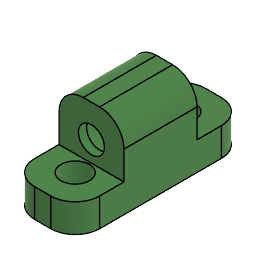
ServoTensioner_v2 (Autodesk Fusion 360 design; units mm, degrees)
Autodesk Fusion 360 part; units mm, degrees
sketch "Sketch1" plane through (0, 0, 0) normal (0, 0, 1) x (1, 0, 0)
  line L0 (0, 6.5) -> (0, -6.5) construction
  circle A0 centre (0, 6.5) radius 1.75
  circle A1 centre (0, -6.5) radius 1.75
  line L1 (4, -4.5) -> (-4, -4.5)
  line L2 (-4, -4.5) -> (-4, 4.5) construction
  line L3 (-4, 4.5) -> (4, 4.5)
  line L4 (4, 4.5) -> (4, -4.5) construction
  line L5 (4, -4.5) -> (-4, 4.5) construction
  line L6 (-4, -4.5) -> (4, 4.5) construction
  line L7 (4, -10.5) -> (-4, -10.5)
  line L8 (-4, -10.5) -> (-4, 10.5)
  line L9 (-4, 10.5) -> (4, 10.5)
  line L10 (4, 10.5) -> (4, -10.5)
  line L11 (4, -10.5) -> (-4, 10.5) construction
  line L12 (-4, -10.5) -> (4, 10.5) construction
  circle A2 centre (0, -6.5) radius 1.4
  circle A3 centre (0, 6.5) radius 1.4
  dimension "d1" = 13
  dimension "d2" = 3.5
  dimension "d3" = 3.5
  dimension "d5" = 9
  dimension "d10" = 2.8
  dimension "d11" = 2.8
  dimension "d14" = 4
  dimension "d15" = 4
  constraint midpoint L0 origin
  constraint vertical L0
  constraint coincident L0.start A0.centre
  constraint coincident L0.end A1.centre
  constraint horizontal L1
  constraint perpendicular L1 L2
  constraint parallel L1 L3
  constraint parallel L2 L4
  constraint coincident L5 origin
  constraint coincident L6 origin
  constraint horizontal L7
  constraint perpendicular L7 L8
  constraint parallel L7 L9
  constraint parallel L8 L10
  constraint coincident L11 origin
  constraint coincident L12 origin
  constraint concentric A1 A2
  constraint concentric A0 A3
  constraint collinear L4 L10
  measures "d1" distance of L0.start L0.end
  measures "d2" diameter of A0
  measures "d3" diameter of A1
  measures "d5" distance of L1.end L2.end
  measures "d10" diameter of A2
  measures "d11" diameter of A3
  measures "d14" distance of L9 L0.start
  measures "d15" distance of L10 L0.start
extrude "Extrude1" add sketch "Sketch1" along normal blind 3.5 contours L1 L7 L8 L10 | L1 L3 L8 L10 | L3 L8 L9 L10
extrude "Extrude2" add sketch "Sketch1" along normal blind 1 contours A0 | A1
extrude "Extrude3" add sketch "Sketch1" along normal blind 10 contours L1 L3 L8 L10
sketch "Sketch2" plane through (0, -4.5, 0) normal (0, -1, 0) x (1, 0, 0)
  line L0 (-4, 3.5) -> (4, 3.5)
  line L1 (4, 3.5) -> (4, 10)
  line L2 (4, 10) -> (-4, 10)
  line L3 (-4, 10) -> (-4, 3.5)
  circle A0 centre (0, 6) radius 2.1
  line L4 (0, 6) -> (0, 3.5)
  circle A1 centre (0, 6) radius 1.6
  dimension "d18" = 4.2
  dimension "d19" = 2.5
  dimension "d24" = 3.2
  constraint coincident A0.centre L4.start
  constraint midpoint L0 L4.end
  constraint perpendicular L0 L4
  constraint concentric A0 A1
  measures "d18" diameter of A0
  measures "d19" distance of A0.centre L4.end
  measures "d24" diameter of A1
extrude "Extrude4" cut sketch "Sketch2" against normal blind 14 contours A0 | A1
fillet "Fillet1" radius 3 2 edges at (-4, 0, 10) (4, 0, 10)
extrude "Extrude5" add sketch "Sketch2" against normal blind 1 contours A0
fillet "Fillet2" radius 3 4 edges at (4, -10.5, 1.75) (-4, -10.5, 1.75) (-4, 10.5, 1.75) (4, 10.5, 1.75)
